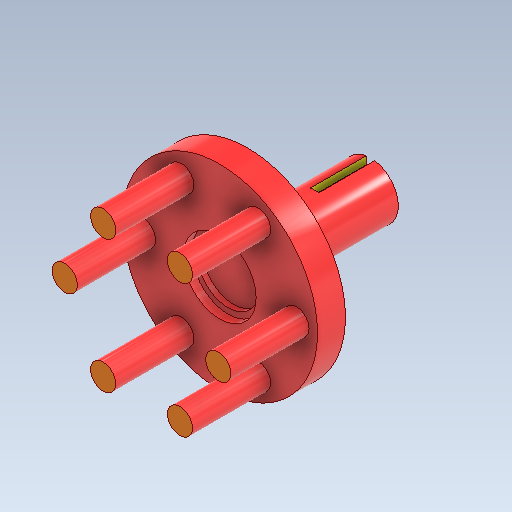
# Autodesk Inventor part: Output Shaft
Saved by Autodesk Inventor 2026.2 (Build 302298010, 298A)
## iProperties
Created: 2026-07-15
Part Number: Output Shaft
Material: Generic
Document SubType Name: Modeling
Designer: maxim
Density: 1 g/cm^3
Appearance: Light Red
Author: maxim
Autodesk Inventor part; units mm, degrees
ref_plane "YZ Plane" through (0, 0, 0) normal (1, 0, 0) x (0, 1, 0)
ref_plane "XZ Plane" through (0, 0, 0) normal (0, 1, 0) x (-1, 0, 0)
ref_plane "XY Plane" through (0, 0, 0) normal (0, 0, 1) x (1, 0, 0)
sketch "Sketch1" plane through (0, 0, 0) normal (0, 0, 1) x (1, 0, 0)
  circle A0 centre (0, 0) radius 27.5 construction
  circle A1 centre (27.5, 0) radius 4.5
  circle A2 centre (13.75, 23.8157) radius 4.5
  circle A3 centre (-13.75, 23.8157) radius 4.5
  circle A4 centre (-27.5, 0) radius 4.5
  circle A5 centre (-13.75, -23.8157) radius 4.5
  circle A6 centre (13.75, -23.8157) radius 4.5
  circle A7 centre (0, 0) radius 35
  circle A8 centre (0, 0) radius 10
  circle A9 centre (0, 0) radius 12.5
  dimension "d0" = 55
  dimension "d1" = 9
  dimension "d4" = 360
  dimension "d6" = 70
  dimension "d11" = 20
  dimension "d19" = 2.5
  constraints: 9 centre point, 4 coincident, 2 horizontal alignment, 15 other
  measures "d1" diameter of A1
  measures "d6" diameter of A7
  measures "d11" diameter of A8
  measures "d19" radial gap between concentric circles of A9 A8
extrude "Extrusion1" add sketch "Sketch1" along normal blind 10 contours A7 | A9
extrude "Extrusion2" add sketch "Sketch1" along normal blind 38 contours A1 | A2 | A3 | A4 | A5 | A6
sketch "Sketch3" plane through (0, 0, 10) normal (0, 0, 1) x (1, 0, 0)
  circle A0 centre (0, 0) radius 10
  circle A1 centre (0, 0) radius 13.025
  circle A2 centre (0, 0) radius 11.025
  dimension "d16" = 20
  dimension "d24" = 26.05
  dimension "d27" = 2
  constraints: 3 centre point, 1 coincident
  measures "d16" diameter of A0
  measures "d24" diameter of A1
  measures "d27" radial gap between concentric circles of A1 A2
extrude "Extrusion4" add sketch "Sketch3" against normal blind 54 contours A0
extrude "Extrusion5" add sketch "Sketch1" against normal blind 2 contours A9
extrude "Extrusion7" cut sketch "Sketch3" against normal blind 5 contours A0 | A2
extrude "Extrusion8" cut sketch "Sketch3" against normal blind 3 contours A1
sketch "Sketch5" plane through (0, 0, -44) normal (0, 0, -1) x (-1, 0, 0)
  circle A0 centre (0, 0) radius 10 projected
  circle A1 centre (0, 0) radius 9.95
  dimension "d30" = 0.05
  constraints: 1 centre point
  measures "d30" radial gap between concentric circles of A0 A1
extrude "Extrusion9" cut sketch "Sketch5" against normal up to surface (42 mm away)
sketch "Sketch6" plane through (0, 0, -44) normal (0, 0, -1) x (-1, 0, 0)
  circle A0 centre (0, 0) radius 9.95 projected
  line L0 (-1.5, 7) -> (1.5, 7)
  line L1 (1.5, 7) -> (1.5, 12)
  line L2 (1.5, 12) -> (-1.5, 12)
  line L3 (-1.5, 12) -> (-1.5, 7)
  dimension "d35" = 1.5
  dimension "d36" = 1.5
  dimension "d38" = 7
  constraints: 8 end point, 2 parallel, 1 horizontal, 1 perpendicular
  measures "d35" distance from line of point (0, 0) L3
  measures "d36" distance from line of L1 point (0, 0)
  measures "d38" distance from line of point (0, 0) L0
extrude "Extrusion10" cut sketch "Sketch6" against normal blind 20 contours L1 L0 L3 A0 | A0 L3 L2 L1 picked at (0.1672, 7.9791)
body "Solid1"
